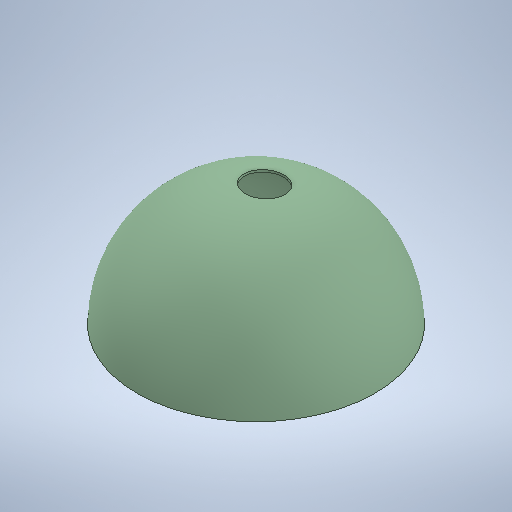
# Autodesk Inventor part: Ball
Saved by Autodesk Inventor 2025 (Build 290162000, 162)
## iProperties
Created: 2024-11-17
Part Number: Ball
Material: Generic
Document SubType Name: Modeling
Designer: ethan
Density: 1 g/cm^3
Appearance: Rubber - Green
Author: ethan
Autodesk Inventor part; units mm, degrees
ref_plane "YZ Plane" through (0, 0, 0) normal (1, 0, 0) x (0, 1, 0)
sketch "Sketch1" plane through (0, 0, 0) normal (0, 1, 0) x (-1, 0, 0)
  line L0 (0, 0) -> (25, 0)
  line L1 (25, 0) -> (25, -25)
  line L2 (25, -25) -> (0, -25)
  line L3 (0, -25) -> (0, 0)
  circle A0 centre (12.5, -12.5) radius 17.6777
  circle A1 centre (12.5, -12.5) radius 21.86
  dimension "d0" = 25
  dimension "d1" = 25
  dimension "d2" = 43.72
  constraints: 8 end point, 2 parallel, 1 centre point, 1 coincident, 1 horizontal, 1 perpendicular, 3 other
  measures "d0" distance of L1.end L2.end
  measures "d1" distance of L0.end L1.end
  measures "d2" diameter of A1
extrude "Extrusion1" add sketch "Sketch1" along normal blind 1 contours L0 L1 L2 L3
ref_plane "Work Plane2" through (0, 0, 0) normal (-0.7071, 0, 0.7071) x (0, 1, 0)
sketch "Sketch3" plane through (0, 0, 0) normal (-0.7071, 0, 0.7071) x (0, 1, 0)
  line L0 (1, 0) -> (1, 17.6777) projected
  line L1 (1, 17.6777) -> (1, 35.3553) projected
  line L2 (1, 17.6777) -> (7.5, 17.6777) construction
  arc A0 (1, 0) -> (1, 35.3553) centre (-19.7885, 17.6777) ccw construction
  circle A1 centre (-19.7885, 17.6777) radius 27.375 construction
  circle A2 centre (-19.7885, 17.6777) radius 27.375
  circle A3 centre (-19.7885, 17.6777) radius 27.875
  line L3 (7.5, 17.6777) -> (8.0865, 17.6777)
  line L4 (-19.7885, 45.0527) -> (-19.7885, 45.5527)
  line L5 (-19.7885, 17.6777) -> (-5.3263, 17.6777)
  line L6 (-19.7885, 17.6777) -> (-19.7885, 45.0527)
  point P0 (0, 0)
  point P1 (7.5865, 17.6777)
  dimension "d10" = 6.5
  dimension "d11" = 54.75
  dimension "d12" = 55.75
  constraints: 10 end point, 7 point on circle, 4 centre point, 3 coincident, 3 horizontal, 1 concentric, 1 perpendicular, 1 vertical
  measures "d10" distance of L0.end L2.end
  measures "d11" diameter of A1
  measures "d12" diameter of A3
revolve "Revolution1" add sketch "Sketch3" angle 360 about axis through (-12.5, -19.7885, -12.5) along (0, 1, 0) picked at (-9.7302, 43.3292) contours A2 L4 A3 L3
ref_plane "Work Plane3" through (0, 1, 0) normal (0, -1, 0) x (1, 0, 0)
sketch "Sketch4" plane through (0, 1, 0) normal (0, -1, 0) x (1, 0, 0)
  line L0 (0, -25) -> (-25, -25) construction
  line L1 (0, 0) -> (0, -25) construction
  line L2 (-25, 0) -> (0, 0) construction
  line L3 (-25, -25) -> (-25, 0) construction
  line L4 (-25, 0) -> (-23, 0) construction
  line L5 (-23, 0) -> (-23, -2) construction
  line L6 (-23, -2) -> (-25, -2) construction
  line L7 (-25, -2) -> (-25, 0) construction
  line L8 (0, 0) -> (-2, 0) construction
  line L9 (-2, 0) -> (-2, -2) construction
  line L10 (-2, -2) -> (0, -2) construction
  line L11 (0, -2) -> (0, 0) construction
  circle A0 centre (-23, -2) radius 1 construction
  circle A1 centre (-23, -2) radius 1
  circle A2 centre (-23, -2) radius 2
  circle A3 centre (-2, -2) radius 1
  circle A4 centre (-2, -2) radius 2
  line L12 (-25, 0) -> (-23, 0) construction
  line L13 (-23, 0) -> (-23, -14.5) construction
  line L14 (-23, -14.5) -> (-25, -14.5) construction
  line L15 (-25, -14.5) -> (-25, 0) construction
  line L16 (0, 0) -> (-2, 0) construction
  line L17 (-2, 0) -> (-2, -14.5) construction
  line L18 (-2, -14.5) -> (0, -14.5) construction
  line L19 (0, -14.5) -> (0, 0) construction
  circle A5 centre (-23, -14.5) radius 1
  circle A6 centre (-2, -14.5) radius 1
  circle A7 centre (-23, -14.5) radius 2
  circle A8 centre (-2, -14.5) radius 2
  dimension "d15" = 2
  dimension "d16" = 2
  dimension "d17" = 2
  dimension "d18" = 2
  dimension "d19" = 2
  dimension "d20" = 4
  dimension "d21" = 2
  dimension "d22" = 4
  dimension "d23" = 2
  dimension "d24" = 14.5
  dimension "d25" = 2
  dimension "d26" = 14.5
  dimension "d27" = 2
  dimension "d28" = 2
  dimension "d29" = 4
  dimension "d30" = 4
  constraints: 32 end point, 9 centre point, 9 coincident, 8 parallel, 4 horizontal, 4 perpendicular, 1 concentric
  measures "d15" distance of L5.end L6.end
  measures "d16" distance of L4.end L5.end
  measures "d17" distance of L10.end L9.end
  measures "d18" distance of L9.end L8.end
  measures "d19" diameter of A0
  measures "d20" diameter of A2
  measures "d21" diameter of A3
  measures "d22" diameter of A4
  measures "d23" distance of L13.end L14.end
  measures "d24" distance of L12.end L13.end
  measures "d25" distance of L18.end L17.end
  measures "d26" distance of L17.end L16.end
  measures "d27" diameter of A5
  measures "d28" diameter of A6
  measures "d29" diameter of A7
  measures "d30" diameter of A8
extrude "Extrusion2" add sketch "Sketch4" against normal up to surface
sketch "Sketch5" plane through (0, 0, 0) normal (0, -1, 0) x (1, 0, 0)
  line L0 (0, -25) -> (-25, -25) construction
  line L1 (0, 0) -> (0, -25) construction
  line L2 (-25, 0) -> (0, 0) construction
  line L3 (-25, -25) -> (-25, 0) construction
  line L4 (-12.5, 0) -> (-12.5, -14.5) construction
  circle A0 centre (-12.5, -14.5) radius 4.5
  dimension "d33" = 14.5
  dimension "d34" = 9
  constraints: 2 end point, 1 centre point, 1 coincident, 1 midpoint, 1 vertical
  measures "d33" distance of L4.start L4.end
  measures "d34" diameter of A0
extrude "Extrusion3" cut sketch "Sketch5" against normal blind 10
sketch "Sketch6" plane through (0, 0, 0) normal (0, -1, 0) x (1, 0, 0)
  circle A0 centre (-12.5, -14.5) radius 4.5 projected
  line L0 (0, -25) -> (-25, -25) projected
  line L1 (0, 0) -> (0, -25) projected
  line L2 (-25, 0) -> (0, 0) projected
  line L3 (-25, -25) -> (-25, 0) projected
extrude "Extrusion4" cut sketch "Sketch6" against normal blind 1
body "Solid1"
